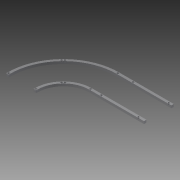
# Autodesk Inventor part: Runner Rails v2
Saved by Autodesk Inventor 2013 (Build 170138000, 138)
## iProperties
Created: 2013-01-15
Part Number: Runner Rails v2
Material: Polycarbonate, Clear
Document SubType Name: Modeling
Designer: actoennies
Mass: 228.775 g
Surface Area: 660.467 cm^2
Volume: 190.646 cm^3
Density: 1.2 g/cm^3
Author: actoennies
Autodesk Inventor part; units mm, degrees
ref_plane "YZ Plane" through (0, 0, 0) normal (1, 0, 0) x (0, 1, 0)
ref_plane "XZ Plane" through (0, 0, 0) normal (0, 1, 0) x (-1, 0, 0)
ref_plane "XY Plane" through (0, 0, 0) normal (0, 0, 1) x (1, 0, 0)
sketch "Sketch1" plane through (0, 0, 0) normal (0, 1, 0) x (-1, 0, 0)
  arc A0 (0, -273.05) -> (273.05, 0) centre (0, 0) ccw
  arc A1 (0, -285.75) -> (285.75, 0) centre (0, 0) ccw
  line L0 (-101.6, -133.35) -> (0, -133.35)
  line L1 (0, -146.05) -> (-101.6, -146.05)
  arc A2 (0, -146.05) -> (146.05, 0) centre (0, 0) ccw
  arc A3 (0, -133.35) -> (133.35, 0) centre (0, 0) ccw
  line L2 (-101.6, -273.05) -> (0, -273.05)
  line L3 (0, -285.75) -> (-101.6, -285.75)
  line L4 (146.05, 0) -> (146.05, 6.35)
  line L5 (133.35, 0) -> (133.35, 6.35)
  line L6 (273.05, 6.35) -> (273.05, 0)
  line L7 (285.75, 6.35) -> (285.75, 0)
  circle A4 centre (103.1708, -94.1906) radius 3.3782
  circle A5 centre (94.1906, -103.1708) radius 3.3782
  circle A6 centre (279.4, 0) radius 3.3782
  circle A7 centre (139.7, 0) radius 3.3782
  circle A8 centre (202.0047, -193.0245) radius 3.3782
  circle A9 centre (193.0245, -202.0047) radius 3.3782
  circle A10 centre (0, -279.4) radius 3.3782
  circle A11 centre (0, -139.7) radius 3.3782
  circle A12 centre (-55.2746, -139.7) radius 3.3782
  circle A13 centre (-78.3684, -279.4) radius 3.3782
  line L8 (285.75, 6.35) -> (273.05, 6.35)
  line L9 (146.05, 6.35) -> (133.35, 6.35)
  line L10 (-101.6, -285.75) -> (-279.4, -285.75)
  line L11 (-279.4, -285.75) -> (-279.4, -273.05)
  line L12 (-279.4, -273.05) -> (-101.6, -273.05)
  line L13 (-101.6, -146.05) -> (-279.4, -146.05)
  line L14 (-279.4, -146.05) -> (-279.4, -133.35)
  line L15 (-279.4, -133.35) -> (-101.6, -133.35)
  dimension "d10" = 12.7
  dimension "d11" = 12.7
  dimension "d13" = 12.7
  dimension "d14" = 6.7564
  dimension "d15" = 6.7564
  dimension "d16" = 6.7564
  dimension "d18" = 6.7564
  dimension "d20" = 6.35
  dimension "d21" = 6.7564
  dimension "d22" = 6.7564
  dimension "d23" = 6.7564
  dimension "d24" = 6.35
  dimension "d26" = 6.7564
  dimension "d27" = 6.35
  dimension "d30" = 6.7564
  dimension "d31" = 6.35
  dimension "d32" = 6.7564
  dimension "d33" = 6.35
  dimension "d50" = 177.8
  dimension "d51" = 177.8
  constraints: 32 end point, 14 centre point, 8 point on circle, 4 parallel, 4 tangent, 3 coincident, 3 collinear, 3 perpendicular
  measures "d10" distance between parallel lines of L4 L5
  measures "d11" distance between parallel lines of L6 L7
  measures "d13" distance of L1.end L0.start
  measures "d14" diameter of A4
  measures "d15" diameter of A5
  measures "d16" diameter of A6
  measures "d18" diameter of A7
  measures "d20" distance from line of L4 A7.centre
  measures "d21" diameter of A8
  measures "d22" diameter of A9
  measures "d23" diameter of A10
  measures "d24" distance from line of L2 A10.centre
  measures "d26" diameter of A11
  measures "d27" distance from line of L0 A11.centre
  measures "d30" diameter of A12
  measures "d31" distance from line of L0 A12.centre
  measures "d32" diameter of A13
  measures "d33" distance from line of L2 A13.centre
  measures "d50" distance of L3.end L10.end
  measures "d51" distance of L14.end L0.start
extrude "Extrusion1" add sketch "Sketch1" along normal blind 12.7
sketch "Sketch2" plane through (0, 12.7, 0) normal (0, 1, 0) x (1, 0, 0)
  circle A0 centre (-279.4, 0) radius 3.3782 projected
  circle A1 centre (0, 279.4) radius 3.3782 projected
  circle A2 centre (78.3684, 279.4) radius 3.3782 projected
  circle A3 centre (-202.0047, 193.0245) radius 3.3782 projected
  circle A4 centre (-193.0245, 202.0047) radius 3.3782 projected
  circle A5 centre (-279.4, 0) radius 4.7625
  circle A6 centre (-202.0047, 193.0245) radius 4.7625
  circle A7 centre (-193.0245, 202.0047) radius 4.7625
  circle A8 centre (0, 279.4) radius 4.7625
  circle A9 centre (78.3684, 279.4) radius 4.7625
  dimension "d36" = 9.525
  dimension "d37" = 9.525
  dimension "d38" = 9.525
  dimension "d39" = 9.525
  dimension "d40" = 9.525
  constraints: 5 centre point, 5 coincident
  measures "d36" diameter of A5
  measures "d37" diameter of A6
  measures "d38" diameter of A7
  measures "d39" diameter of A8
  measures "d40" diameter of A9
extrude "Extrusion2" cut sketch "Sketch2" against normal blind 6.35 contours A0 | A1 | A2 | A3 | A4 | A5 | A6 | A7 | A8 | A9
sketch "Sketch3" plane through (0, 12.7, 0) normal (0, 1, 0) x (1, 0, 0)
  circle A0 centre (-139.7, 0) radius 3.3782 projected
  circle A1 centre (-103.1708, 94.1906) radius 3.3782 projected
  circle A2 centre (-94.1906, 103.1708) radius 3.3782 projected
  circle A3 centre (55.2746, 139.7) radius 3.3782 projected
  circle A4 centre (0, 139.7) radius 3.3782 projected
  circle A5 centre (-139.7, 0) radius 4.7625
  circle A6 centre (-103.1708, 94.1906) radius 4.7625
  circle A7 centre (-94.1906, 103.1708) radius 4.7625
  circle A8 centre (0, 139.7) radius 4.7625
  circle A9 centre (55.2746, 139.7) radius 4.7625
  dimension "d43" = 9.525
  dimension "d44" = 9.525
  dimension "d45" = 9.525
  dimension "d46" = 9.525
  dimension "d47" = 9.525
  constraints: 5 centre point, 5 coincident
  measures "d43" diameter of A5
  measures "d44" diameter of A6
  measures "d45" diameter of A7
  measures "d46" diameter of A8
  measures "d47" diameter of A9
extrude "Extrusion3" cut sketch "Sketch3" against normal blind 6.35 contours A0 | A1 | A2 | A3 | A4 | A5 | A6 | A7 | A8 | A9
sketch "Sketch4" plane through (0, 0, 0) normal (0, -1, 0) x (1, 0, 0)
  circle A0 centre (-139.7, 0) radius 3.3782 projected
  circle A1 centre (-103.1708, -94.1906) radius 3.3782 projected
  circle A2 centre (-94.1906, -103.1708) radius 3.3782 projected
  circle A3 centre (55.2746, -139.7) radius 3.3782 projected
  circle A4 centre (0, -139.7) radius 3.3782 projected
  line L0 (279.4, -133.35) -> (0, -133.35) projected
  arc A5 (-133.35, 0) -> (0, -133.35) centre (0, 0) ccw projected
  line L1 (-133.35, 0) -> (-133.35, 6.35) projected
  line L2 (-133.35, 6.35) -> (-146.05, 6.35) projected
  line L3 (-146.05, 6.35) -> (-146.05, 0) projected
  arc A6 (-146.05, 0) -> (0, -146.05) centre (0, 0) ccw projected
  line L4 (0, -146.05) -> (279.4, -146.05) projected
  line L5 (279.4, -146.05) -> (279.4, -133.35) projected
  line L6 (274.32, -191.0842) -> (264.16, -191.0842) projected
  line L7 (264.16, -191.0842) -> (264.16, -181.5592) projected
  line L8 (264.16, -181.5592) -> (274.32, -181.5592) projected
  line L9 (274.32, -181.5592) -> (274.32, -191.0842) projected
  line L10 (279.4, -224.79) -> (264.16, -197.4342) projected
  line L11 (264.16, -197.4342) -> (279.4, -197.4342) projected
  line L12 (279.4, -173.99) -> (279.4, -197.4342) projected
  line L13 (279.4, -173.99) -> (264.16, -173.99) projected
  line L14 (264.16, -173.99) -> (264.16, -154.675) projected
  arc A7 (264.16, -154.675) -> (116.84, -55.9994) centre (110.49, -224.79) ccw projected
  line L15 (116.84, -63.5) -> (116.84, -55.9994) projected
  line L16 (102.87, -63.5) -> (116.84, -63.5) projected
  line L17 (102.87, -73.66) -> (102.87, -63.5) projected
  line L18 (116.84, -73.66) -> (102.87, -73.66) projected
  line L19 (116.84, -78.8781) -> (116.84, -73.66) projected
  arc A8 (116.84, -370.7019) -> (116.84, -78.8781) centre (110.49, -224.79) ccw projected
  line L20 (116.84, -375.92) -> (116.84, -370.7019) projected
  line L21 (102.87, -375.92) -> (116.84, -375.92) projected
  line L22 (102.87, -386.08) -> (102.87, -375.92) projected
  line L23 (116.84, -386.08) -> (102.87, -386.08) projected
  line L24 (116.84, -393.5806) -> (116.84, -386.08) projected
  arc A9 (116.84, -393.5806) -> (279.4, -224.79) centre (110.49, -224.79) ccw projected
  line L25 (101.6, 53.8711) -> (101.6, -411.5586) projected
  circle A10 centre (101.6, -224.79) radius 158.75
  circle A11 centre (112.2452, -224.79) radius 157.48 construction
  circle A12 centre (259.9533, -279.4) radius 3.3782
  circle A13 centre (244.758, -139.7) radius 3.3782
  circle A14 centre (259.9533, -279.4) radius 3.3782 projected
  circle A15 centre (244.758, -139.7) radius 3.3782 projected
  point P0 (110.49, -224.79)
  dimension "d61" = 314.96
  dimension "d62" = 6.7564
  dimension "d63" = 6.7564
  constraints: 4 centre point, 2 point on circle, 1 point on line
  measures "d61" diameter of A11
  measures "d62" diameter of A12
  measures "d63" diameter of A13
extrude "Extrusion5" cut sketch "Sketch4" against normal blind 25.4 contours A12 | A13
body "Solid1"
